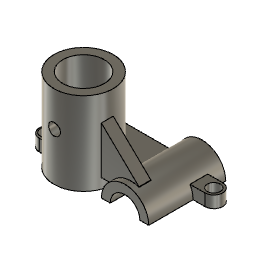
drawing_3 v3 (Autodesk Fusion 360 design; units mm, degrees)
Autodesk Fusion 360 part; units mm, degrees
sketch "Sketch1" plane through (0, 0, 0) normal (0, 0, 1) x (1, 0, 0)
  circle A0 centre (0, 0) radius 10
  circle A1 centre (0, 0) radius 6.25
  line L0 (-9.9999, -0.0411) -> (-6.2499, -0.0411)
  line L1 (6.2499, -0.0363) -> (9.9999, -0.0363)
  line L2 (-6.2499, -0.0411) -> (6.2499, -0.0363)
  dimension "d2" = 20
  dimension "d3" = 12.5
  constraint coincident A0.centre A1.centre
  constraint coincident A0 L0.start
  constraint coincident A1 L0.end
  constraint horizontal L0
  constraint coincident A1 L1.start
  constraint coincident A0 L1.end
  constraint parallel L0 L1
  measures "d2" diameter of A0
  measures "d3" diameter of A1
extrude "Extrude1" add sketch "Sketch1" along normal blind 65 contours A0 A1 L0 L1 picked at (-8.6933, 0.7678) makes body 1
sketch "Sketch2" plane through (0, -0.0411, 0) normal (0, -1, 0) x (1, 0, 0)
  line L0 (-9.9999, 0) -> (-6.2499, 0)
  line L1 (-6.2499, 0) -> (-6.2499, 65)
  line L2 (-6.2499, 65) -> (-9.9999, 65)
  line L3 (-9.9999, 65) -> (-9.9999, 0)
  line L4 (-50, 10) -> (-9.9999, 10)
  circle A0 centre (-50, 50) radius 17.5
  circle A1 centre (-50, 50) radius 25
  line L5 (-50, 10) -> (-62, 10)
  line L6 (-62, 10) -> (-62, 28.0683)
  line L7 (-50, 50) -> (-80, 50)
  circle A2 centre (-80, 50) radius 5.5
  circle A3 centre (-80, 50) radius 7.5
  line L8 (-79.9683, 57.4999) -> (-79.9683, 55.4999)
  line L9 (-79.9683, 50.0001) -> (-79.9683, 44.5001)
  line L10 (-79.9683, 44.5001) -> (-79.9683, 42.5001)
  line L11 (-80, 50) -> (-79.9683, 55.4999)
  line L12 (-79.9683, 57.4999) -> (-73.8566, 57.4741)
  line L13 (-79.9683, 42.5001) -> (-73.8566, 42.5259)
  line L14 (-50, 50) -> (-9.9999, 50)
  line L15 (-9.9999, 10) -> (-9.9999, 50)
  circle A4 centre (30, 20) radius 5.5
  circle A5 centre (30, 20) radius 7.5
  line L16 (30, 20) -> (30, 14.5)
  line L17 (30, 20) -> (30, 25.5)
  line L18 (30, 27.5) -> (10, 27.5)
  line L19 (30, 14.5) -> (30, 12.5)
  line L20 (30, 12.5) -> (10, 12.5)
  line L21 (10, 12.5) -> (10, 27.5)
  dimension "d10" = 35
  dimension "d11" = 50
  dimension "d15" = 11
  dimension "d16" = 15
  dimension "d19" = 11
  dimension "d20" = 15
  constraint concentric A0 A1
  constraint parallel L4 L5
  constraint coincident A1 L6.end
  constraint perpendicular L5 L6
  constraint coincident A0.centre A1.centre
  constraint horizontal L7
  constraint coincident L7.end A2.centre
  constraint concentric A2 A3
  constraint coincident A3 L8.start
  constraint coincident A2 L8.end
  constraint vertical L8
  constraint coincident A2 L9.end
  constraint parallel L8 L9
  constraint coincident A3 L10.end
  constraint parallel L9 L10
  constraint coincident A1 L12.end
  constraint tangent A3 L12
  constraint coincident A1 L13.end
  constraint tangent A3 L13
  constraint coincident L3 L14.end
  constraint perpendicular L3 L14
  constraint perpendicular L14 L15
  constraint concentric A4 A5
  constraint coincident A4.centre A5.centre
  constraint coincident A4 L16.end
  constraint vertical L16
  constraint coincident A4 L17.end
  constraint parallel L16 L17
  constraint coincident A5 L18.start
  constraint tangent A5 L18
  constraint perpendicular L17 L18
  constraint coincident A5 L19.end
  constraint parallel L16 L19
  constraint tangent A5 L20
  constraint perpendicular L20 L21
  measures "d10" diameter of A0
  measures "d11" diameter of A1
  measures "d15" diameter of A2
  measures "d16" diameter of A3
  measures "d19" diameter of A4
  measures "d20" diameter of A5
sketch "Sketch3" plane through (0, 0, 0) normal (0, 0, 1) x (1, 0, 0)
  circle A0 centre (0, 0) radius 20
  circle A1 centre (0, 0) radius 12.5
  line L0 (-20, -0.0287) -> (-12.5, -0.0287)
  line L1 (0, 0) -> (12.5, 0)
  line L2 (20, 0) -> (12.5, 0)
  dimension "d21" = 40
  dimension "d22" = 25
  constraint coincident A0.centre A1.centre
  constraint concentric A0 A1
  constraint coincident A0 L0.start
  constraint horizontal L0
  constraint coincident A1 L1.end
  constraint parallel L0 L1
  constraint coincident A0 L2.start
  constraint parallel L1 L2
  measures "d21" diameter of A0
  measures "d22" diameter of A1
extrude "Extrude2" add sketch "Sketch3" along normal blind 65 separate body contours A0 A1 L0 L2 | A0 A1 L0 L2 makes body 2
extrude "Extrude3" add sketch "Sketch2" against normal blind 10 contours L3 L4 A1 L5 L6 L14 L15 | A0 A1 L7 A3 L14 | A0 A1 L7 A3 L14 | A1 A3 L12 | A1 L7 A2 A3 | A1 A2 A3 L8 | A2 A3 L8 L10 | A1 A3 L13 | A1 L7 A2 A3 | A1 A2 A3 L10 | A5 | A5 L18 L20 L21 bodies 1 2
sketch "Sketch4" plane through (0, 0, 0) normal (0, 0, -1) x (1, 0, 0)
  circle A0 centre (0, 0) radius 12.5
  circle A1 centre (0, 0) radius 20
  circle A2 centre (0, 0) radius 12.5
  constraint coincident A0.centre A1.centre
extrude "Extrude4" cut sketch "Sketch4" against normal blind 85 contours A0 A2 bodies 1
sketch "Sketch5" plane through (0, 0, 65) normal (0, 0, 1) x (-1, 0, 0)
  circle A0 centre (0, 0) radius 12.5
  circle A1 centre (0, 0) radius 20
  line L0 (20, -0.0045) -> (12.5, -0.0045)
  line L1 (12.5, -0.0045) -> (-12.5, -0.0045)
  line L2 (-12.5, -0.0045) -> (-20, -0.0045)
  line L3 (-20, 20) -> (-20, -0.0045)
  line L4 (-20, 20) -> (14, 22)
  line L5 (14, 22) -> (20, 13)
  line L6 (20, 13) -> (20, -0.0045)
  constraint coincident A1 L0.start
  constraint coincident A0 L0.end
  constraint horizontal L0
  constraint coincident A0 L1.end
  constraint parallel L0 L1
  constraint coincident A1 L2.end
  constraint parallel L1 L2
  constraint perpendicular L2 L3
extrude "Extrude5" cut sketch "Sketch5" against normal blind 85 contours A0 L1 | A0 L0 L2 L3 L4 L5 L6 picked at (3.0541, 2.8328) bodies 1
move_body "Move1" bodies 1 to x (1, 0, 0) y (0, 0, 1) z (0, -1, 0) at (0, 31.0373, 31.1196)
sketch "Sketch6" plane through (0, 0, 0) normal (0, 0, 1) x (1, 0, 0)
  circle A0 centre (-81, -19) radius 5.5
  dimension "d31" = 11
  measures "d31" diameter of A0
extrude "Extrude6" cut sketch "Sketch6" along normal blind 55 bodies 1
sketch "Sketch7" plane through (0, 0, 41.0785) normal (0, 0, 1) x (-1, 0, 0)
  arc A0 (80.7044, 13.5079) -> (80.2956, 24.4547) centre (81, 19) ccw
  arc A1 (80.2956, 24.4547) -> (80.7044, 13.5079) centre (80, 18.9627) ccw
  line L0 (17.3442, 18.9627) -> (17.3442, -21.0373)
  line L1 (17.3442, -21.0373) -> (62, -21.0373)
  line L2 (62, -21.0373) -> (62, -2.9691)
  arc A2 (62, -2.9691) -> (73.8566, 11.4885) centre (50, 18.9627) ccw
  line L3 (73.8566, 11.4885) -> (79.9683, 11.4627)
  arc A3 (79.9683, 11.4627) -> (79.9683, 26.4626) centre (80, 18.9627) ccw
  line L4 (79.9683, 26.4626) -> (73.8566, 26.4368)
  arc A4 (73.8566, 26.4368) -> (25, 18.9627) centre (50, 18.9627) ccw
  line L5 (25, 18.9627) -> (17.3442, 18.9627)
  circle A5 centre (50, 18.9627) radius 17.5
  circle A6 centre (81, 19) radius 5.5
  circle A7 centre (80, 18.9627) radius 5.5
  constraint concentric A0 A6
  constraint concentric A1 A7
extrude "Extrude7" add sketch "Sketch7" along normal blind 4.5 separate body contours A1 A6 A7 makes body 3
sketch "Sketch8" plane through (-0.0499, -11.8004, 0) normal (0.004225, 0.999991, 0) x (-0.999991, 0.004225, 0)
  line L0 (73.8074, 31.0785) -> (79.9192, 31.0785)
  line L1 (79.9192, 31.0785) -> (79.9192, 41.0785)
  line L2 (79.9192, 41.0785) -> (73.8074, 41.0785)
  line L3 (73.8074, 41.0785) -> (73.8074, 31.0785)
  line L4 (73.8074, 41.0785) -> (81.6473, 41.0785)
  line L5 (81.6473, 41.0785) -> (81.6473, 46.5121)
  line L6 (81.6473, 46.5121) -> (73.8074, 46.5121)
  line L7 (73.8074, 46.5121) -> (73.8074, 41.0785)
  constraint horizontal L4
  constraint vertical L5
  constraint horizontal L6
  constraint vertical L7
  constraint coincident L2.end L3.start
extrude "Extrude8" add 1 faces at (-74.9038, -19.7733, 45.5785) along direction (0, 0, -1) blind 14.5 on bodies 3 bodies 3 1
extrude "Extrude9" cut sketch "Sketch8" against normal blind 54 contours L2 L4 L5 L6 L7 bodies 3
sketch "Sketch9" plane through (0, 0, 41.0785) normal (0, 0, 1) x (-1, 0, 0)
  circle A0 centre (81, 19) radius 5.5
  circle A1 centre (50, 18.9627) radius 17.5
  line L0 (79.9683, 26.4626) -> (73.8566, 26.4368)
  arc A2 (73.8566, 26.4368) -> (25, 18.9627) centre (50, 18.9627) ccw
  line L1 (25, 18.9627) -> (17.3442, 18.9627)
  line L2 (17.3442, 18.9627) -> (17.3442, -21.0373)
  line L3 (17.3442, -21.0373) -> (62, -21.0373)
  line L4 (62, -21.0373) -> (62, -2.9691)
  arc A3 (62, -2.9691) -> (73.8566, 11.4885) centre (50, 18.9627) ccw
  line L5 (73.8566, 11.4885) -> (79.9683, 11.4627)
  arc A4 (79.9683, 11.4627) -> (79.9683, 26.4626) centre (80, 18.9627) ccw
  circle A5 centre (50, 18.9627) radius 17.5
  circle A6 centre (50, 18.9627) radius 25
  dimension "d40" = 50
  constraint concentric A1 A5
  constraint concentric A5 A6
  measures "d40" diameter of A6
extrude "Extrude10" add sketch "Sketch9" along normal blind 60 contours A2 A3 A6 bodies 3
sketch "Sketch10" plane through (0, -18.9627, 0) normal (0, -1, 0) x (1, 0, 0)
  line L0 (-20, 31.0785) -> (-20, 31.1196)
  arc A0 (-20, 31.1241) -> (-20, 31.1196) centre (0, 31.1196) ccw
  arc A1 (-17.3442, 41.0785) -> (-20, 31.1241) centre (0, 31.1196) ccw
  line L1 (-17.3442, 41.0785) -> (-25, 41.0785)
  line L2 (-25, 41.0785) -> (-25, 31.0785)
  line L3 (-25, 31.0785) -> (-20, 31.0785)
  line L4 (-25, 41.0785) -> (18, 41.0785)
  line L5 (12.5332, 41.0785) -> (12.5332, 61.0785)
  line L6 (-25, 101) -> (-25, 81)
  line L7 (7, 50) -> (-7, 50)
  line L8 (-25, 81) -> (7, 50)
  line L9 (-7, 50) -> (-17.3442, 41.0785)
  line L10 (-25, 41.0785) -> (-25, 81)
  dimension "d43" = 20
  dimension "d44" = 20
  constraint coincident L1.end L2.start
  constraint perpendicular L2 L4
  constraint coincident L4 L5.start
  constraint perpendicular L4 L5
  constraint vertical L6
  constraint horizontal L7
  constraint coincident A1.start L1.start
  measures "d43" distance of L5.start L5.end
  measures "d44" distance of L6.start L6.end
extrude "Extrude11" add sketch "Sketch10" along normal blind 10 contours L1 L4 L7 L8 L9 L10 bodies 3
sketch "Sketch11" plane through (0, -18.9627, 0) normal (0, 1, 0) x (-1, 0, 0)
  arc A0 (6.5976, 50) -> (-6.5976, 50) centre (0, 31.1196) ccw
  line L0 (6.5976, 50) -> (7, 50)
  line L1 (7, 50) -> (7.3033, 49.7384)
  arc A1 (17.3442, 41.0785) -> (7.3033, 49.7384) centre (0, 31.1196) ccw
  line L2 (17.3442, 41.0785) -> (25, 41.0785)
  line L3 (25, 41.0785) -> (25, 81)
  line L4 (25, 81) -> (-7, 50)
  line L5 (-7, 50) -> (-6.5976, 50)
  line L6 (75, 100) -> (50, 100)
  line L7 (50, 100) -> (50, 31.446)
  line L8 (50, 31.446) -> (54, 31.446)
  line L9 (54, 31.446) -> (54, 71.446)
  line L10 (54, 71.446) -> (50, 71.446)
  circle A2 centre (50, 71.446) radius 5
  dimension "d47" = 40
  dimension "d48" = 10
  constraint horizontal L6
  constraint perpendicular L6 L7
  constraint perpendicular L7 L8
  constraint perpendicular L6 L9
  constraint coincident L7 L10.end
  constraint perpendicular L7 L10
  constraint coincident L10.end A2.centre
  measures "d47" distance of L8.end L9.end
  measures "d48" diameter of A2
extrude "Extrude12" cut sketch "Sketch11" along normal mid plane 130 contours L7 L9 L10 A2 | L7 A2 | L7 L9 L10 A2 bodies 3
